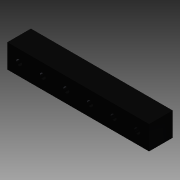
# Autodesk Inventor part: Main Header
Saved by Autodesk Inventor 2013 (Build 170138000, 138)
## iProperties
Created: 2013-07-31
Part Number: Main Header
Material: ABS Plastic
Document SubType Name: Modeling
Designer: Kyle
Density: 1 g/cm^3
Author: Kyle
Autodesk Inventor part; units mm, degrees
ref_plane "YZ Plane" through (0, 0, 0) normal (1, 0, 0) x (0, 1, 0)
ref_plane "XZ Plane" through (0, 0, 0) normal (0, 1, 0) x (-1, 0, 0)
ref_plane "XY Plane" through (0, 0, 0) normal (0, 0, 1) x (1, 0, 0)
sketch "Sketch1" plane through (0, 0, 0) normal (0, 0, 1) x (1, 0, 0)
  line L0 (0, 0) -> (15.24, 0)
  line L1 (15.24, 0) -> (15.24, -2.54)
  line L2 (15.24, -2.54) -> (0, -2.54)
  line L3 (0, -2.54) -> (0, 0)
  dimension "d0" = 15.24
  dimension "d1" = 2.54
  constraints: 8 end point, 2 parallel, 1 horizontal, 1 perpendicular
  measures "d0" distance of L0.start L0.end
  measures "d1" distance of L2.end L0.start
extrude "Extrusion1" add sketch "Sketch1" along normal blind 2.54
sketch "Sketch2" plane through (0, 0, 2.54) normal (0, 0, 1) x (1, 0, 0)
  line L0 (15.24, 0) -> (0, 0) projected
  line L1 (0, 0) -> (0, -2.54) projected
  circle A0 centre (1.27, -1.27) radius 0.3175
  circle A1 centre (3.81, -1.27) radius 0.3175
  circle A2 centre (6.35, -1.27) radius 0.3175
  circle A3 centre (8.89, -1.27) radius 0.3175
  circle A4 centre (11.43, -1.27) radius 0.3175
  circle A5 centre (13.97, -1.27) radius 0.3175
  dimension "d4" = 0.635
  dimension "d6" = 1.27
  dimension "d9" = 2.54
  constraints: 6 centre point, 1 horizontal, 10 other
  measures "d4" diameter of A0
  measures "d6" distance from line of L1 A0.centre
  measures "d9" distance of A0.centre A1.centre
extrude "Extrusion2" cut sketch "Sketch2" against normal blind 2.54
body "Solid1"
